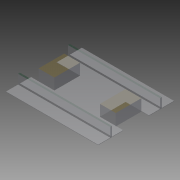
# Autodesk Inventor part: eboard
Saved by Autodesk Inventor 2014 (Build 180170000, 170)
## iProperties
Created: 2014-01-10
Part Number: eboard
Material: Generic
Document SubType Name: Modeling
Designer: pc
Density: 1 g/cm^3
Appearance: Polycarbonate - Clear
Author: pc
Autodesk Inventor part; units mm, degrees
ref_plane "YZ Plane" through (0, 0, 0) normal (1, 0, 0) x (0, 1, 0)
ref_plane "XZ Plane" through (0, 0, 0) normal (0, 1, 0) x (-1, 0, 0)
ref_plane "XY Plane" through (0, 0, 0) normal (0, 0, 1) x (1, 0, 0)
sketch "Sketch1" plane through (0, 0, 0) normal (0, 1, 0) x (-1, 0, 0)
  line L0 (0, 0) -> (628.65, 0)
  line L1 (628.65, 0) -> (628.65, 518.16)
  line L2 (628.65, 518.16) -> (0, 518.16)
  line L3 (0, 518.16) -> (0, 0)
  line L4 (0, 346.71) -> (50.8, 346.71)
  line L5 (50.8, 346.71) -> (50.8, 171.45)
  line L6 (50.8, 171.45) -> (0, 171.45)
  line L7 (0, 171.45) -> (0, 346.71)
  line L8 (628.65, 346.71) -> (577.85, 346.71)
  line L9 (577.85, 346.71) -> (577.85, 171.45)
  line L10 (577.85, 171.45) -> (628.65, 171.45)
  line L11 (628.65, 171.45) -> (628.65, 346.71)
  dimension "d0" = 628.65
  dimension "d1" = 518.16
  dimension "d2" = 50.8
  dimension "d3" = 50.8
  dimension "d4" = 171.45
  dimension "d5" = 171.45
  dimension "d6" = 171.45
  dimension "d7" = 171.45
  constraints: 24 end point, 6 parallel, 3 horizontal, 3 perpendicular, 2 point on line
  measures "d0" distance of L2.end L1.end
  measures "d1" distance of L1.end L0.end
  measures "d2" distance of L4.start L4.end
  measures "d3" distance of L8.start L8.end
  measures "d4" distance between parallel lines of L2 L4
  measures "d5" distance between parallel lines of L0 L6
  measures "d6" distance between parallel lines of L0 L10
  measures "d7" distance from line of L2 L8.end
extrude "Extrusion1" add sketch "Sketch1" along normal blind 3.048 contours L3 L6 L5 L4 L2 L1 L8 L9 L10 L0
sketch "Sketch2" plane through (0, 3.048, 0) normal (0, 1, 0) x (1, 0, 0)
  line L0 (-577.85, -171.45) -> (-469.9, -171.45)
  line L1 (-469.9, -171.45) -> (-469.9, -346.71)
  line L2 (-469.9, -346.71) -> (-577.85, -346.71)
  line L3 (-577.85, -346.71) -> (-577.85, -171.45)
  line L4 (-50.8, -346.71) -> (-158.75, -346.71)
  line L5 (-158.75, -346.71) -> (-158.75, -171.45)
  line L6 (-158.75, -171.45) -> (-50.8, -171.45)
  line L7 (-50.8, -171.45) -> (-50.8, -346.71)
  dimension "d10" = 107.95
  dimension "d11" = 107.95
  constraints: 16 end point, 4 parallel, 2 horizontal, 2 perpendicular
  measures "d10" distance of L1.end L2.end
  measures "d11" distance of L5.end L6.end
extrude "Extrusion3" add sketch "Sketch2" along normal blind 76.2
sketch "Sketch3" plane through (0, 3.048, 0) normal (0, 1, 0) x (1, 0, 0)
  line L0 (-628.65, -346.71) -> (-628.65, -518.16) projected
  line L1 (0, -518.16) -> (0, -346.71) projected
  line L2 (-50.8, -346.71) -> (-158.75, -346.71) projected
  line L3 (0, -171.45) -> (0, 0) projected
  line L4 (-628.65, 0) -> (-628.65, -171.45) projected
  line L5 (-577.85, -171.45) -> (-469.9, -171.45) projected
  line L6 (-628.65, -422.91) -> (0, -422.91)
  line L7 (0, -422.91) -> (0, -435.61)
  line L8 (0, -435.61) -> (-628.65, -435.61)
  line L9 (-628.65, -435.61) -> (-628.65, -422.91)
  line L10 (-628.65, -82.55) -> (0, -82.55)
  line L11 (0, -82.55) -> (0, -95.25)
  line L12 (0, -95.25) -> (-628.65, -95.25)
  line L13 (-628.65, -95.25) -> (-628.65, -82.55)
  dimension "d16" = 12.7
  dimension "d17" = 12.7
  dimension "d18" = 76.2
  dimension "d19" = 76.2
  constraints: 16 end point, 4 parallel, 4 point on line, 2 horizontal, 2 perpendicular
  measures "d16" distance of L6.end L7.end
  measures "d17" distance of L10.end L11.end
  measures "d18" distance between parallel lines of L5 L12
  measures "d19" distance between parallel lines of L2 L6
extrude "Extrusion4" add sketch "Sketch3" along normal blind 63.5
equation "\"d3\" = d2"
equation "\"d5\" = d4"
equation "\"d6\" = d4"
equation "\"d7\" = d4"
body "Solid1"
